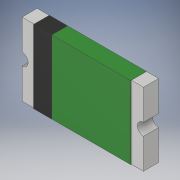
# Autodesk Inventor part: fuse
Saved by Autodesk Inventor 2019 (Build 230136000, 136)
## iProperties
Created: 2019-03-13
Part Number: fuse
Material: Generico
Document SubType Name: Modeling
Designer: Thartarus
Density: 1 g/cm^3
Appearance: Default
Author: Thartarus
Autodesk Inventor part; units mm, degrees
ref_plane "YZ Plane" through (0, 0, 0) normal (1, 0, 0) x (0, 1, 0)
ref_plane "XZ Plane" through (0, 0, 0) normal (0, 1, 0) x (-1, 0, 0)
ref_plane "XY Plane" through (0, 0, 0) normal (0, 0, 1) x (1, 0, 0)
sketch "Schizzo1" plane through (0, 0, 0) normal (0, 0, 1) x (1, 0, 0)
  line L0 (-1, 0.6) -> (1, 0.6)
  line L1 (1, 0.6) -> (1, -0.6) construction
  line L2 (1, -0.6) -> (-1, -0.6)
  line L3 (-1, -0.6) -> (-1, 0.6) construction
  arc A0 (-1, -0.1) -> (-1, 0.1) centre (-1, 0) ccw
  line L4 (-1, 0.6) -> (-1, 0.1)
  line L5 (-1, -0.1) -> (-1, -0.6)
  arc A1 (1, 0.1) -> (1, -0.1) centre (1, 0) ccw
  line L6 (1, -0.1) -> (1, -0.6)
  line L7 (1, 0.1) -> (1, 0.6)
  line L8 (-0.8, 0.6) -> (0.8, 0.6)
  line L9 (0.8, 0.6) -> (0.8, -0.6)
  line L10 (0.8, -0.6) -> (-0.8, -0.6)
  line L11 (-0.8, -0.6) -> (-0.8, 0.6)
  point P0 (0, 0)
  dimension "d0" = 2
  dimension "d1" = 1.2
  dimension "d2" = 1
  dimension "d3" = 0.6
  dimension "d4" = 0.1
  dimension "d5" = 0.6
  dimension "d6" = 0.1
  dimension "d7" = 0.2
  dimension "d8" = 0.2
  constraints: 24 end point, 6 point on line, 4 collinear, 4 parallel, 4 point on circle, 2 centre point, 2 horizontal, 2 midpoint, 2 perpendicular, 1 coincident
  measures "d0" distance of L1.end L2.end
  measures "d1" distance of L0.end L1.end
  measures "d2" distance from line of point (0, 0) L1
  measures "d3" distance from line of point (0, 0) L2
  measures "d4" radius of A0
  measures "d5" distance from line of L2 A0.centre
  measures "d6" radius of A1
  measures "d7" distance between parallel lines of L3 L11
  measures "d8" distance between parallel lines of L7 L9
extrude "Estrusione1" add sketch "Schizzo1" along normal blind 0.25
sketch "Schizzo2" plane through (0, 0, 0.25) normal (0, 0, 1) x (1, 0, 0)
  line L0 (1, 0.6) -> (-1, 0.6) projected
  line L1 (-1, -0.6) -> (1, -0.6) projected
  line L2 (-0.8, 0.6) -> (0.8, 0.6)
  line L3 (0.8, 0.6) -> (0.8, -0.6)
  line L4 (0.8, -0.6) -> (-0.8, -0.6)
  line L5 (-0.8, -0.6) -> (-0.8, 0.6)
  line L6 (1, 0.1) -> (1, 0.6) projected
  line L7 (-1, 0.6) -> (-1, 0.1) projected
  point P0 (0, 0)
  dimension "d11" = 0.2
  dimension "d12" = 0.2
  constraints: 8 end point, 2 parallel, 2 point on line, 1 horizontal, 1 perpendicular
  measures "d11" distance between parallel lines of L6 L3
  measures "d12" distance between parallel lines of L7 L5
extrude "Estrusione2" add sketch "Schizzo2" along normal blind 0.01
sketch "Schizzo3" plane through (0, 0, 0.26) normal (0, 0, 1) x (1, 0, 0)
  line L0 (-0.8, -0.6) -> (-0.8, 0.6) projected
  line L1 (-1, -0.6) -> (1, -0.6) projected
  line L2 (-0.8, 0.6) -> (-0.5, 0.6)
  line L3 (-0.5, 0.6) -> (-0.5, -0.6)
  line L4 (-0.5, -0.6) -> (-0.8, -0.6)
  line L5 (-0.8, -0.6) -> (-0.8, 0.6)
  point P0 (0, 0)
  dimension "d15" = 0.3
  constraints: 8 end point, 2 parallel, 1 horizontal, 1 perpendicular, 1 point on line
  measures "d15" distance between parallel lines of L0 L3
extrude "Estrusione3" add sketch "Schizzo3" along normal blind 0.001
sketch "Schizzo4" plane through (-1, 0.6, 0) normal (0, 1, 0) x (1, 0, 0)
  line L0 (1.8, -0.25) -> (1.8, -0.26) projected
  line L1 (2, 0) -> (0, 0) projected
  line L2 (1.8, -0.25) -> (2, -0.25)
  line L3 (2, -0.25) -> (2, 0)
  line L4 (2, 0) -> (1.8, 0)
  line L5 (1.8, 0) -> (1.8, -0.25)
  line L6 (0, 0) -> (0.2, 0)
  line L7 (0.2, 0) -> (0.2, -0.25)
  line L8 (0.2, -0.25) -> (0, -0.25)
  line L9 (0, -0.25) -> (0, 0)
  point P0 (1, 0)
  constraints: 16 end point, 4 parallel, 2 horizontal, 2 perpendicular
extrude "Estrusione4" cut sketch "Schizzo4" against normal blind 0.001
sketch "Schizzo5" plane through (-1, -0.6, 0) normal (0, -1, 0) x (1, 0, 0)
  line L0 (0.2, 0.25) -> (0.2, 0.261) projected
  line L1 (0.2, 0.25) -> (0, 0.25)
  line L2 (0, 0.25) -> (0, 0)
  line L3 (0, 0) -> (0.2, 0)
  line L4 (0.2, 0) -> (0.2, 0.25)
  line L5 (1.8, 0.25) -> (2, 0.25) projected
  line L6 (0, 0) -> (2, 0) projected
  line L7 (1.8, 0.25) -> (2, 0.25)
  line L8 (2, 0.25) -> (2, 0)
  line L9 (2, 0) -> (1.8, 0)
  line L10 (1.8, 0) -> (1.8, 0.25)
  point P0 (1, 0)
  constraints: 16 end point, 4 parallel, 2 horizontal, 2 perpendicular
extrude "Estrusione5" cut sketch "Schizzo5" against normal blind 0.001
sketch "Schizzo7" plane through (-0.8, -0.6, 0) normal (0, -1, 0) x (1, 0, 0)
  line L0 (0.3, 0.261) -> (0, 0.261) projected
  line L1 (0, 0.261) -> (0, 0) projected
  line L2 (0.3, 0.261) -> (0, 0.261)
  line L3 (0, 0.261) -> (0, 0)
  line L4 (0, 0) -> (0.3, 0)
  line L5 (0.3, 0) -> (0.3, 0.261)
  point P0 (0.8, 0)
  constraints: 8 end point, 2 parallel, 1 horizontal, 1 perpendicular
extrude "Estrusione6" add sketch "Schizzo7" along normal blind 0.001
sketch "Schizzo8" plane through (-0.8, 0.6, 0) normal (0, 1, 0) x (1, 0, 0)
  line L0 (0.3, -0.261) -> (0, -0.261) projected
  line L1 (0, -0.261) -> (0.3, -0.261)
  line L2 (0.3, -0.261) -> (0.3, 0)
  line L3 (0.3, 0) -> (0, 0)
  line L4 (0, 0) -> (0, -0.261)
  line L5 (0.3, -0.26) -> (0.3, -0.261) projected
  point P0 (0.8, 0)
  constraints: 8 end point, 2 parallel, 1 collinear, 1 horizontal, 1 perpendicular
extrude "Estrusione7" add sketch "Schizzo8" along normal blind 0.001
